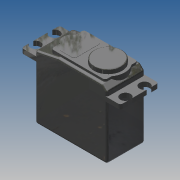
# Autodesk Inventor part: HS-225MG
Saved by Autodesk Inventor 2012 SP2 (Build 160219200, 219)
## iProperties
Created: 2013-05-18
Part Number: HS-225MG
Document SubType Name: Modeling
Designer: Holger
Density: 1 g/cm^3
Material: Standard
Author: Holger
Autodesk Inventor part; units mm, degrees
ref_plane "YZ Plane" through (0, 0, 0) normal (1, 0, 0) x (0, 1, 0)
ref_plane "XZ Plane" through (0, 0, 0) normal (0, 1, 0) x (-1, 0, 0)
ref_plane "XY Plane" through (0, 0, 0) normal (0, 0, 1) x (1, 0, 0)
sketch "Skizze1" plane through (0, 0, 0) normal (0, 0, 1) x (1, 0, 0)
  line L0 (-16, 8.5) -> (16, 8.5)
  line L1 (16, 8.5) -> (16, -8.5)
  line L2 (16, -8.5) -> (-16, -8.5)
  line L3 (-16, -8.5) -> (-16, 8.5)
  point P0 (0, 0)
  dimension "d0" = 32
  dimension "d1" = 17
  dimension "d2" = 8.5
  dimension "d3" = 16
  constraints: 8 end point, 2 parallel, 1 horizontal, 1 perpendicular
  measures "d0" distance of L1.end L2.end
  measures "d1" distance of L0.end L1.end
  measures "d2" distance from line of L2 point (0, 0)
  measures "d3" distance from line of point (0, 0) L3
extrude "Extrusion1" add sketch "Skizze1" along normal blind 30
sketch "Skizze2" plane through (0, 0, 30) normal (0, 0, 1) x (1, 0, 0)
  line L0 (16, 8.5) -> (16, -8.5) projected
  circle A0 centre (8, 0) radius 6.25
  point P0 (0, 0)
  dimension "d6" = 12.5
  dimension "d7" = 8
  constraints: 1 centre point
  measures "d6" diameter of A0
  measures "d7" distance from line of A0.centre L0
extrude "Extrusion2" add sketch "Skizze2" along normal blind 3
sketch "Skizze6" plane through (16, -8.5, 0) normal (1, 0, 0) x (0, 0, -1)
  line L0 (0, 0) -> (-30, 0) projected
  line L1 (0, 17) -> (0, 0) projected
  line L2 (0, 17) -> (-30, 17) projected
  line L3 (-26, 0) -> (-24, 0)
  line L4 (-24, 0) -> (-24, 17)
  line L5 (-24, 17) -> (-26, 17)
  line L6 (-26, 17) -> (-26, 0)
  point P0 (0, 8.5)
  dimension "d33" = 2
  dimension "d34" = 24
  constraints: 8 end point, 2 parallel, 2 point on line, 1 horizontal, 1 perpendicular
  measures "d33" distance of L4.end L5.end
  measures "d34" distance between parallel lines of L1 L4
extrude "Extrusion6" add sketch "Skizze6" along normal blind 6 contours L0 L6 L2 L4
sketch "Skizze7" plane through (-16, -8.5, 0) normal (-1, 0, 0) x (0, 0, 1)
  line L0 (0, 17) -> (30, 17) projected
  line L1 (0, 0) -> (0, 17) projected
  line L2 (0, 0) -> (30, 0) projected
  line L3 (26, 17) -> (24, 17)
  line L4 (24, 17) -> (24, 0)
  line L5 (24, 0) -> (26, 0)
  line L6 (26, 0) -> (26, 17)
  point P0 (0, 8.5)
  dimension "d37" = 2
  dimension "d38" = 24
  constraints: 8 end point, 2 parallel, 2 point on line, 1 horizontal, 1 perpendicular
  measures "d37" distance of L4.end L5.end
  measures "d38" distance between parallel lines of L1 L4
extrude "Extrusion7" add sketch "Skizze7" along normal blind 6 contours L0 L6 L2 L4
sketch "Skizze8" plane through (-16, -8.5, 26) normal (0, 0, 1) x (1, 0, 0)
  line L0 (0, 0) -> (-6, 0) projected
  line L1 (0, 17) -> (0, 0) projected
  line L2 (0, 17) -> (-6, 17) projected
  circle A0 centre (-4, 12.75) radius 2.25
  circle A1 centre (-4, 4.25) radius 2.25
  point P0 (16, 8.5)
  dimension "d41" = 4.5
  dimension "d42" = 4.5
  dimension "d43" = 4
  dimension "d44" = 4
  dimension "d45" = 4.25
  dimension "d46" = 4.25
  constraints: 2 centre point
  measures "d41" diameter of A0
  measures "d42" diameter of A1
  measures "d43" distance from line of L1 A0.centre
  measures "d44" distance from line of L1 A1.centre
  measures "d45" distance from line of L0 A1.centre
  measures "d46" distance from line of L2 A0.centre
extrude "Extrusion8" cut sketch "Skizze8" against normal blind 2
sketch "Skizze9" plane through (16, -8.5, 26) normal (0, 0, 1) x (1, 0, 0)
  line L0 (0, 17) -> (6, 17) projected
  line L1 (0, 0) -> (0, 17) projected
  line L2 (0, 0) -> (6, 0) projected
  circle A0 centre (4, 12.75) radius 2.25
  circle A1 centre (4, 4.25) radius 2.25
  point P0 (-16, 8.5)
  dimension "d49" = 4.5
  dimension "d50" = 4.5
  dimension "d51" = 4.25
  dimension "d52" = 4.25
  dimension "d53" = 4
  dimension "d54" = 4
  constraints: 2 centre point
  measures "d49" diameter of A0
  measures "d50" diameter of A1
  measures "d51" distance from line of L0 A0.centre
  measures "d52" distance from line of L2 A1.centre
  measures "d53" distance from line of L1 A1.centre
  measures "d54" distance from line of L1 A0.centre
extrude "Extrusion9" cut sketch "Skizze9" against normal blind 2
sketch "Skizze10" plane through (0, 0, 30) normal (0, 0, 1) x (1, 0, 0)
  circle A0 centre (8, 0) radius 6.25 projected
  line L0 (-16, 8.5) -> (16, 8.5) projected
  line L1 (-10, 7.25) -> (14, 7.25)
  line L2 (14, -7.25) -> (-10, -7.25)
  arc A1 (-10, 3.4411) -> (-10, -3.4411) centre (-8.0397, 0) ccw
  line L3 (-10, -7.25) -> (-10, -3.4411)
  line L4 (-10, 3.4411) -> (-10, 7.25)
  arc A2 (14, -4.4512) -> (14, 4.4512) centre (8, 0) ccw
  line L5 (14, 7.25) -> (14, 4.4512)
  line L6 (14, -4.4512) -> (14, -7.25)
  point P0 (0, 0)
  dimension "d58" = 14.5
  dimension "d59" = 24
  dimension "d61" = 1.25
  constraints: 12 end point, 5 parallel, 4 point on circle, 2 centre point, 2 perpendicular, 1 coincident, 1 horizontal
  measures "d58" distance of L2.end L1.start
  measures "d59" distance of L1.start L1.end
  measures "d61" distance between parallel lines of L0 L1
extrude "Extrusion10" add sketch "Skizze10" along normal blind 1
chamfer "Fase1" distance 2 distance2 10 1 edges at (-16, 0, 30) measured on face at (-16, 0, 29.5)
chamfer "Fase2" distance 2 distance2 2 1 edges at (16, 0, 30) measured on face at (16, 0, 29.5)
fillet "Rundung2" radius 1 4 edges at (-10, -7.25, 30.1) (14, -7.25, 30.5) (-10, 7.25, 30.1) (14, 7.25, 30.5)
fillet "Rundung3" radius 1 24 edges at (4, 8.5, 30) (-11, 8.5, 29) (-16, 8.5, 27) (-16, 8.5, 12) (0, 8.5, 0) (16, 8.5, 12) (16, 8.5, 27) (15, 8.5, 29) (-16, 0, 28) (-16, 0, 0) (-16, -8.5, 12) (-16, -8.5, 27) (-11, -8.5, 29) (4, -8.5, 30) (15, -8.5, 29) (16, -8.5, 27) (16, -8.5, 12) (0, -8.5, 0) (16, 0, 28) (16, 0, 0) (22, -8.5, 25) (22, 8.5, 25) (-22, -8.5, 25) (-22, 8.5, 25)
sketch "Skizze11" plane through (0, 0, 31) normal (0, 0, 1) x (1, 0, 0)
  line L0 (-10, 3.4411) -> (-10, 6.25) projected
  line L1 (-7, 6) -> (-2, 6)
  line L2 (-1, 5) -> (-1, -5)
  line L3 (-2, -6) -> (-7, -6)
  line L4 (-8, -5) -> (-8, 5)
  line L5 (-5.901, 8.5) -> (-15, 8.5) projected
  arc A0 (-7, 6) -> (-8, 5) centre (-7, 5) ccw
  arc A1 (-1, 5) -> (-2, 6) centre (-2, 5) ccw
  arc A2 (-2, -6) -> (-1, -5) centre (-2, -5) ccw
  arc A3 (-8, -5) -> (-7, -6) centre (-7, -5) ccw
  point P0 (0, 0)
  dimension "d73" = 12
  dimension "d74" = 7
  dimension "d75" = 2.5
  dimension "d76" = 2
  dimension "d77" = 1
  constraints: 8 end point, 8 point on circle, 8 tangent, 4 centre point, 3 equal radius, 2 parallel, 1 horizontal, 1 perpendicular
  measures "d73" distance between parallel lines of L3 L1
  measures "d74" distance between parallel lines of L2 L4
  measures "d75" distance between parallel lines of L5 L1
  measures "d76" distance between parallel lines of L4 L0
  measures "d77" radius of A0
extrude "Extrusion11" add sketch "Skizze11" along normal blind 0.1
fillet "Rundung4" radius 0.5 1 edges at (1.75, 0, 33)
equation "\"d2\" = 0.5 * d1"
equation "\"d3\" = 0.5 * d0"
